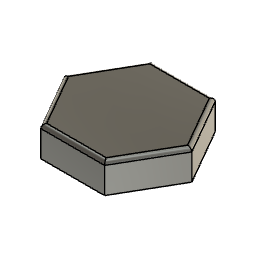
Mirror-v02 v1 (Autodesk Fusion 360 design; units mm, degrees)
Autodesk Fusion 360 part; units mm, degrees
sketch "Skizze1" plane through (0, 0, 0) normal (0, 0, 1) x (1, 0, 0)
  line L0 (-2.1362, 3.7) -> (-4.2724, 0)
  line L1 (-4.2724, 0) -> (-2.1362, -3.7)
  line L2 (-2.1362, -3.7) -> (2.1362, -3.7)
  line L3 (2.1362, -3.7) -> (4.2724, 0)
  line L4 (4.2724, 0) -> (2.1362, 3.7)
  line L5 (2.1362, 3.7) -> (-2.1362, 3.7)
  dimension "d1" = 7.4
  measures "d1" distance of L2 L5
extrude "Extrusion1" add sketch "Skizze1" along normal blind 2
fillet "Abrundung1" radius 0.25 1 faces at (-0.7121, -1.2333, 2)
